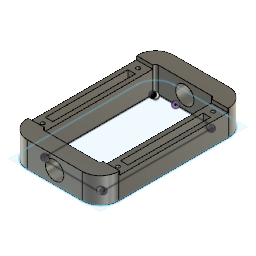
rotor v2 (Autodesk Fusion 360 design; units mm, degrees)
Autodesk Fusion 360 part; units mm, degrees
note: some values were not read from the file. Set by a fixed rule: which sketch regions a step uses.
sketch "Sketch1" plane through (0, 0, 0) normal (0, 0, 1) x (1, 0, 0)
  line L0 (0, 0) -> (50, 0)
  line L1 (50, 0) -> (50, 80)
  line L2 (50, 80) -> (0, 80)
  line L3 (0, 80) -> (0, 0)
  line L4 (9, 9) -> (41, 9)
  line L5 (41, 9) -> (41, 71)
  line L6 (41, 71) -> (9, 71)
  line L7 (9, 71) -> (9, 9)
  line L8 (2, 62.5) -> (7, 62.5)
  line L9 (7, 62.5) -> (7, 17.5)
  line L10 (7, 17.5) -> (2, 17.5)
  line L11 (2, 17.5) -> (2, 62.5)
  line L12 (0, 40) -> (2, 40)
  line L13 (25, 71) -> (25, 60)
  line L14 (48, 62.5) -> (43, 62.5)
  line L15 (48, 17.5) -> (48, 62.5)
  line L16 (43, 62.5) -> (43, 17.5)
  line L17 (43, 17.5) -> (48, 17.5)
  dimension "d1" = 50
  dimension "d2" = 80
  dimension "d3" = -9
  dimension "d4" = 45
  dimension "d5" = 90
  dimension "d6" = 2
  dimension "d7" = 5
  constraint horizontal L0
  constraint vertical L1
  constraint horizontal L2
  constraint vertical L3
  constraint coincident L0.start L3.end
  constraint horizontal L8
  constraint vertical L9
  constraint horizontal L10
  constraint vertical L11
  constraint midpoint L3 L12.start
  constraint midpoint L11 L12.end
  constraint midpoint L6 L13.start
  constraint perpendicular L6 L13
  constraint symmetric L8.start L13 L14.start
  constraint symmetric L8.end L13 L14.end
  constraint symmetric L9.end L13 L16.end
  constraint symmetric L10.end L13 L15.start
  measures "d1" distance of L1.end L2.end
  measures "d2" distance of L0.end L1.end
  measures "d4" distance of L8.start L10.end
  measures "d5" angle of L3 L12
  measures "d6" distance of L12.start L12.end
  measures "d7" distance of L8.start L8.end
extrude "Extrude1" add sketch "Sketch1" along normal blind 10
sketch "Sketch2" plane through (0, 0, 0) normal (0, 0, -1) x (1, 0, 0)
  line L0 (2, -17.5) -> (7, -17.5)
  line L1 (7, -17.5) -> (7, -62.5)
  line L2 (7, -62.5) -> (2, -62.5)
  line L3 (2, -62.5) -> (2, -17.5)
  line L4 (43, -17.5) -> (48, -17.5)
  line L5 (48, -17.5) -> (48, -62.5)
  line L6 (48, -62.5) -> (43, -62.5)
  line L7 (43, -62.5) -> (43, -17.5)
  line L8 (9, -71) -> (9, -9)
  line L9 (9, -9) -> (41, -9)
  line L10 (41, -9) -> (41, -71)
  line L11 (41, -71) -> (9, -71)
  line L12 (0, 0) -> (0, -80)
  line L13 (0, -80) -> (50, -80)
  line L14 (50, -80) -> (50, 0)
  line L15 (50, 0) -> (0, 0)
  line L16 (0, 0) -> (50, 0)
  line L17 (50, 0) -> (50, -80)
  line L18 (50, -80) -> (0, -80)
  line L19 (0, -80) -> (0, 0)
  constraint horizontal L16
  constraint vertical L17
  constraint horizontal L18
  constraint vertical L19
  constraint coincident L13.end L14.start
  constraint coincident L12.start L15.end
extrude "Extrude2" add sketch "Sketch2" along normal blind 2 contours L0 L1 L2 L3 | L4 L5 L6 L7 | L12 L13 L14 L15 L16 L17 L18 L19
sketch "Sketch3" plane through (0, 0, 10) normal (0, 0, 1) x (-1, 0, 0)
  line L0 (-7, -17.5) -> (-2, -17.5)
  line L1 (-2, -17.5) -> (-2, -62.5)
  line L2 (-2, -62.5) -> (-7, -62.5)
  line L3 (-7, -62.5) -> (-7, -17.5)
  line L4 (-9, -9) -> (-9, -71)
  line L5 (-9, -71) -> (-41, -71)
  line L6 (-41, -71) -> (-41, -9)
  line L7 (-41, -9) -> (-9, -9)
  line L8 (-48, -17.5) -> (-43, -17.5)
  line L9 (-43, -17.5) -> (-43, -62.5)
  line L10 (-43, -62.5) -> (-48, -62.5)
  line L11 (-48, -62.5) -> (-48, -17.5)
  line L12 (0, -80) -> (0, 0)
  line L13 (0, 0) -> (-50, 0)
  line L14 (-50, 0) -> (-50, -80)
  line L15 (-50, -80) -> (0, -80)
  line L16 (0, -80) -> (-50, -80)
  line L17 (-50, -80) -> (-50, 0)
  line L18 (-50, 0) -> (0, 0)
  line L19 (0, 0) -> (0, -80)
  line L20 (0, -10.5) -> (-50, -10.5)
  line L21 (-50, -10.5) -> (-50, -69.5)
  line L22 (-50, -69.5) -> (0, -69.5)
  line L23 (0, -69.5) -> (0, -10.5)
  line L24 (-4.5, -17.5) -> (-4.5, -10.5)
  line L25 (-4.5, -62.5) -> (-4.5, -69.5)
  line L26 (-45.5, -62.5) -> (-45.5, -69.5)
  line L27 (-45.5, -17.5) -> (-45.5, -10.5)
  circle A0 centre (-4.5, -14) radius 1
  circle A1 centre (-45.5, -14) radius 1
  circle A2 centre (-45.5, -66) radius 1
  circle A3 centre (-4.5, -66) radius 1
  dimension "d12" = 7
  dimension "d13" = 7
  dimension "d14" = 2
  dimension "d15" = 2
  dimension "d16" = 2
  dimension "d17" = 2
  constraint horizontal L16
  constraint vertical L17
  constraint horizontal L18
  constraint vertical L19
  constraint coincident L13.end L14.start
  constraint coincident L12.start L15.end
  constraint horizontal L20
  constraint vertical L21
  constraint horizontal L22
  constraint vertical L23
  constraint coincident L14 L21.end
  constraint coincident L12 L20.start
  constraint midpoint L0 L24.start
  constraint coincident L20 L24.end
  constraint perpendicular L20 L24
  constraint midpoint L2 L25.start
  constraint coincident L22 L25.end
  constraint perpendicular L22 L25
  constraint midpoint L10 L26.start
  constraint coincident L22 L26.end
  constraint perpendicular L22 L26
  constraint midpoint L8 L27.start
  constraint coincident L20 L27.end
  constraint perpendicular L20 L27
  constraint midpoint L24 A0.centre
  constraint midpoint L27 A1.centre
  constraint midpoint L26 A2.centre
  constraint midpoint L25 A3.centre
  measures "d12" distance of L0 L20
  measures "d13" distance of L2 L22
  measures "d14" diameter of A3
  measures "d15" diameter of A2
  measures "d16" diameter of A1
  measures "d17" diameter of A0
extrude "Extrude3" cut sketch "Sketch3" against normal blind 10 contours L24 A0 | L24 A0 | L25 A3 | L25 A3 | L27 A1 | L27 A1 | L26 A2 | L26 A2
extrude "Extrude4" add sketch "Sketch3" along normal blind 2 contours L4 L6 L7 L12 L13 L14 L17 L18 L19 L20 | L4 L5 L6 L12 L14 L15 L16 L17 L19 L22
sketch "Sketch4" plane through (0, 0, 0) normal (0, -1, 0) x (1, 0, 0)
  line L0 (50, -2) -> (50, 12)
  line L1 (50, 12) -> (0, 12)
  line L2 (0, 12) -> (0, -2)
  line L3 (0, -2) -> (50, -2)
  line L4 (25, 12) -> (25, -2)
  circle A0 centre (25, 5) radius 5
  dimension "d22" = 10
  constraint midpoint L1 L4.start
  constraint midpoint L3 L4.end
  constraint midpoint L4 A0.centre
  measures "d22" diameter of A0
extrude "Extrude5" cut sketch "Sketch4" against normal blind 100 contours L4 A0 | L4 A0
sketch "Sketch5" plane through (0, 0, -2) normal (0, 0, -1) x (1, 0, 0)
  line L0 (41, -9) -> (41, -71)
  line L1 (41, -71) -> (9, -71)
  line L2 (9, -71) -> (9, -9)
  line L3 (9, -9) -> (41, -9)
  line L4 (0, -80) -> (50, -80)
  line L5 (50, -80) -> (50, 0)
  line L6 (50, 0) -> (0, 0)
  line L7 (0, 0) -> (0, -80)
  line L8 (10, -80) -> (40, -80)
  line L9 (50, -70) -> (50, -10)
  line L10 (40, 0) -> (10, 0)
  line L11 (0, -10) -> (0, -70)
  line L12 (39.5, -9) -> (10.5, -9)
  line L13 (9, -10.5) -> (9, -69.5)
  line L14 (10.5, -71) -> (39.5, -71)
  line L15 (41, -69.5) -> (41, -10.5)
  arc A0 (10.5, -9) -> (9, -10.5) centre (10.5, -10.5) ccw
  arc A1 (41, -10.5) -> (39.5, -9) centre (39.5, -10.5) ccw
  arc A2 (9, -69.5) -> (10.5, -71) centre (10.5, -69.5) ccw
  arc A3 (39.5, -71) -> (41, -69.5) centre (39.5, -69.5) ccw
  arc A4 (10, 0) -> (0, -10) centre (10, -10) ccw
  arc A5 (50, -10) -> (40, 0) centre (40, -10) ccw
  arc A6 (0, -70) -> (10, -80) centre (10, -70) ccw
  arc A7 (40, -80) -> (50, -70) centre (40, -70) ccw
  point P0 (20, -71)
  point P1 (9, -10.5)
  point P2 (41, -10.5)
  point P3 (41, -69.5)
  point P4 (9, -69.5)
  dimension "d29" = 10
  dimension "d30" = 10
  dimension "d31" = 10
  dimension "d32" = 10
  constraint horizontal L8
  constraint vertical L9
  constraint horizontal L10
  constraint vertical L11
  constraint horizontal L12
  constraint vertical L13
  constraint horizontal L14
  constraint vertical L15
  constraint tangent L12 A0
  constraint tangent L13 A0
  constraint tangent L12 A1
  constraint tangent L15 A1
  constraint tangent L13 A2
  constraint tangent L14 A2
  constraint tangent L14 A3
  constraint tangent L15 A3
  constraint tangent L10 A4
  constraint tangent L11 A4
  constraint tangent L9 A5
  constraint tangent L10 A5
  constraint tangent L8 A6
  constraint tangent L11 A6
  constraint tangent L8 A7
  constraint tangent L9 A7
  constraint coincident L14 P0
  constraint collinear L0 L15
  constraint collinear L3 L12
  constraint collinear L2 L13
  constraint coincident P1 L13.start
  constraint coincident P2 L15.end
  constraint coincident P3 L15.start
  constraint coincident P4 L13.end
  measures "d29" radius of A4
  measures "d30" radius of A5
  measures "d31" radius of A6
  measures "d32" radius of A7
extrude "Extrude6" cut sketch "Sketch5" against normal blind 100 contours L4 L7 A6 | L4 L5 A7 | L6 L7 A4 | L5 L6 A5
extrude "Extrude7" add sketch "Sketch5" against normal up to surface (14 mm away) contours L0 L3 A1 | L0 L1 A3 | L2 L3 A0 | L1 L2 A2
extrude "Extrude8" add 1 faces at (48, 32.5, 3.3333) along direction (-1, 0, 0) blind 0.5
extrude "Extrude9" add 1 faces at (7, 47.5, 3.3333) along direction (-1, 0, 0) blind 0.5
extrude "Extrude10" add 1 faces at (2, 32.5, 3.3333) along direction (1, 0, 0) blind 0.5
extrude "Extrude11" add 1 faces at (43, 47.5, 3.3333) along direction (1, 0, 0) blind 0.5
